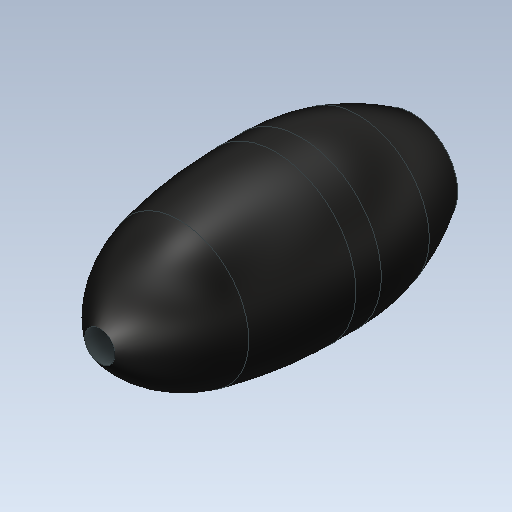
# Autodesk Inventor part: sail_weight
Saved by Autodesk Inventor 2020 (Build 240168000, 168)
## iProperties
Created: 2017-12-03
Part Number: sail_weight
Material: Lead
Document SubType Name: Modeling
Designer: stedrock
Density: 11.34 g/cm^3
Appearance: Lead
Mass: 409.157 g
Surface Area: 57.3985 cm^2
Volume: 36.0808 cm^3
Author: stedrock
Autodesk Inventor part; units mm, degrees
ref_plane "YZ Plane" through (0, 0, 0) normal (1, 0, 0) x (0, 1, 0)
ref_plane "XZ Plane" through (0, 0, 0) normal (0, 1, 0) x (-1, 0, 0)
ref_plane "XY Plane" through (0, 0, 0) normal (0, 0, 1) x (1, 0, 0)
sketch "Sketch1" plane through (0, 0, 0) normal (1, 0, 0) x (0, 1, 0)
  line L0 (0, 0) -> (0, 63)
  line L1 (0, 0) -> (9, 0)
  line L2 (15.9, 22) -> (15.9, 27)
  arc A0 (14.1466, 10.7593) -> (15.9, 22) centre (-21.0068, 22) ccw
  arc A1 (9, 0) -> (14.1466, 10.7593) centre (-27.5407, 24.0893) ccw
  arc A2 (15.9, 27) -> (15.9, 27) centre (-40077.1724, 27) ccw
  arc A3 (15.9, 27) -> (13.7227, 45.9678) centre (-67.8106, 27) ccw
  arc A4 (13.7227, 45.9678) -> (1.5995, 62.5596) centre (-11.8275, 40.0238) ccw
  arc A5 (1.5995, 62.5596) -> (0, 63) centre (0, 59.875) ccw
  dimension "d0" = 63
  dimension "d1" = 9
  dimension "d2" = 15.9
  dimension "d4" = 5
  dimension "d5" = 22
  constraints: 12 point on circle, 6 centre point, 6 end point, 6 tangent, 2 vertical, 1 horizontal, 1 line through centre, 1 point on line
  measures "d0" distance of L0.start L0.end
  measures "d1" distance of L0.start L1.end
  measures "d2" distance between parallel lines of L0 L2
  measures "d4" distance of L2.start L2.end
  measures "d5" distance from line of L1 L2.start
revolve "Revolution1" add sketch "Sketch1" angle 360 about axis through (0, 0, 0) along (0, 0, 1) contours L0 A5 A4 A3 L2 A0 A1 L1
sketch "Sketch2" plane through (0, 0, 0) normal (0, 0, 1) x (1, 0, 0)
  circle A0 centre (0, 0) radius 3
  dimension "d6" = 6
  constraints: 1 centre point, 1 coincident
  measures "d6" diameter of A0
extrude "hole" cut sketch "Sketch2" along normal through all
shell "Shell1" [suppressed]
split "Split1" [suppressed]
sketch "ribs" plane through (0, 0, 0) normal (1, 0, 0) x (0, 1, 0)
  line L0 (0, 0) -> (0, 68.6975) construction
  line L1 (0, 0) -> (23.2714, 0) construction
  line L2 (-0.6, 80.4959) -> (0.6, 80.4959)
  line L3 (0.6, 80.4959) -> (0.6, -19.5041)
  line L4 (0.6, -19.5041) -> (-0.6, -19.5041)
  line L5 (-0.6, -19.5041) -> (-0.6, 80.4959)
  line L6 (-0.6, 80.4959) -> (0.6, -19.5041) construction
  line L7 (0.6, 80.4959) -> (-0.6, -19.5041) construction
  line L8 (0, 0) -> (0, -28.2792) construction
  line L9 (-21.2582, -13.3041) -> (21.2582, -13.3041)
  line L10 (21.2582, -13.3041) -> (21.2582, -14.5041)
  line L11 (21.2582, -14.5041) -> (-21.2582, -14.5041)
  line L12 (-21.2582, -14.5041) -> (-21.2582, -13.3041)
  line L13 (-21.2582, -13.3041) -> (21.2582, -14.5041) construction
  line L14 (21.2582, -13.3041) -> (-21.2582, -14.5041) construction
  line L15 (0, 0) -> (34.6426, 0) construction
  line L16 (9.4, 80.4959) -> (10.6, 80.4959)
  line L17 (10.6, -19.5041) -> (9.4, -19.5041)
  line L18 (10, 0) -> (10, -28.2792) construction
  line L19 (10.6, 80.4959) -> (10.6, -19.5041)
  line L20 (9.4, -19.5041) -> (9.4, 80.4959)
  line L21 (9.4, 80.4959) -> (10.6, -19.5041) construction
  line L22 (10.6, 80.4959) -> (9.4, -19.5041) construction
  line L23 (19.4, 80.4959) -> (20.6, 80.4959)
  line L24 (20.6, -19.5041) -> (19.4, -19.5041)
  line L25 (20, 0) -> (20, -28.2792) construction
  line L26 (20.6, 80.4959) -> (20.6, -19.5041)
  line L27 (19.4, -19.5041) -> (19.4, 80.4959)
  line L28 (19.4, 80.4959) -> (20.6, -19.5041) construction
  line L29 (20.6, 80.4959) -> (19.4, -19.5041) construction
  line L30 (29.4, 80.4959) -> (30.6, 80.4959)
  line L31 (30.6, -19.5041) -> (29.4, -19.5041)
  line L32 (30, 0) -> (30, -28.2792) construction
  line L33 (30.6, 80.4959) -> (30.6, -19.5041)
  line L34 (29.4, -19.5041) -> (29.4, 80.4959)
  line L35 (29.4, 80.4959) -> (30.6, -19.5041) construction
  line L36 (30.6, 80.4959) -> (29.4, -19.5041) construction
  line L37 (39.4, 80.4959) -> (40.6, 80.4959)
  line L38 (40.6, -19.5041) -> (39.4, -19.5041)
  line L39 (40, 0) -> (40, -28.2792) construction
  line L40 (40.6, 80.4959) -> (40.6, -19.5041)
  line L41 (39.4, -19.5041) -> (39.4, 80.4959)
  line L42 (39.4, 80.4959) -> (40.6, -19.5041) construction
  line L43 (40.6, 80.4959) -> (39.4, -19.5041) construction
  line L44 (21.2582, -3.3041) -> (21.2582, -4.5041)
  line L45 (21.2582, -4.5041) -> (-21.2582, -4.5041)
  line L46 (-21.2582, -3.3041) -> (21.2582, -3.3041)
  line L47 (-21.2582, -3.3041) -> (21.2582, -4.5041) construction
  line L48 (21.2582, -3.3041) -> (-21.2582, -4.5041) construction
  line L49 (-21.2582, -4.5041) -> (-21.2582, -3.3041)
  line L50 (21.2582, 6.6959) -> (21.2582, 5.4959)
  line L51 (21.2582, 5.4959) -> (-21.2582, 5.4959)
  line L52 (-21.2582, 6.6959) -> (21.2582, 6.6959)
  line L53 (-21.2582, 6.6959) -> (21.2582, 5.4959) construction
  line L54 (21.2582, 6.6959) -> (-21.2582, 5.4959) construction
  line L55 (-21.2582, 5.4959) -> (-21.2582, 6.6959)
  line L56 (21.2582, 16.6959) -> (21.2582, 15.4959)
  line L57 (21.2582, 15.4959) -> (-21.2582, 15.4959)
  line L58 (-21.2582, 16.6959) -> (21.2582, 16.6959)
  line L59 (-21.2582, 16.6959) -> (21.2582, 15.4959) construction
  line L60 (21.2582, 16.6959) -> (-21.2582, 15.4959) construction
  line L61 (-21.2582, 15.4959) -> (-21.2582, 16.6959)
  line L62 (21.2582, 26.6959) -> (21.2582, 25.4959)
  line L63 (21.2582, 25.4959) -> (-21.2582, 25.4959)
  line L64 (-21.2582, 26.6959) -> (21.2582, 26.6959)
  line L65 (-21.2582, 26.6959) -> (21.2582, 25.4959) construction
  line L66 (21.2582, 26.6959) -> (-21.2582, 25.4959) construction
  line L67 (-21.2582, 25.4959) -> (-21.2582, 26.6959)
  line L68 (21.2582, 36.6959) -> (21.2582, 35.4959)
  line L69 (21.2582, 35.4959) -> (-21.2582, 35.4959)
  line L70 (-21.2582, 36.6959) -> (21.2582, 36.6959)
  line L71 (-21.2582, 36.6959) -> (21.2582, 35.4959) construction
  line L72 (21.2582, 36.6959) -> (-21.2582, 35.4959) construction
  line L73 (-21.2582, 35.4959) -> (-21.2582, 36.6959)
  line L74 (21.2582, 46.6959) -> (21.2582, 45.4959)
  line L75 (21.2582, 45.4959) -> (-21.2582, 45.4959)
  line L76 (-21.2582, 46.6959) -> (21.2582, 46.6959)
  line L77 (-21.2582, 46.6959) -> (21.2582, 45.4959) construction
  line L78 (21.2582, 46.6959) -> (-21.2582, 45.4959) construction
  line L79 (-21.2582, 45.4959) -> (-21.2582, 46.6959)
  line L80 (21.2582, 56.6959) -> (21.2582, 55.4959)
  line L81 (21.2582, 55.4959) -> (-21.2582, 55.4959)
  line L82 (-21.2582, 56.6959) -> (21.2582, 56.6959)
  line L83 (-21.2582, 56.6959) -> (21.2582, 55.4959) construction
  line L84 (21.2582, 56.6959) -> (-21.2582, 55.4959) construction
  line L85 (-21.2582, 55.4959) -> (-21.2582, 56.6959)
  line L86 (21.2582, 66.6959) -> (21.2582, 65.4959)
  line L87 (21.2582, 65.4959) -> (-21.2582, 65.4959)
  line L88 (-21.2582, 66.6959) -> (21.2582, 66.6959)
  line L89 (-21.2582, 66.6959) -> (21.2582, 65.4959) construction
  line L90 (21.2582, 66.6959) -> (-21.2582, 65.4959) construction
  line L91 (-21.2582, 65.4959) -> (-21.2582, 66.6959)
  line L92 (21.2582, 76.6959) -> (21.2582, 75.4959)
  line L93 (21.2582, 75.4959) -> (-21.2582, 75.4959)
  line L94 (-21.2582, 76.6959) -> (21.2582, 76.6959)
  line L95 (-21.2582, 76.6959) -> (21.2582, 75.4959) construction
  line L96 (21.2582, 76.6959) -> (-21.2582, 75.4959) construction
  line L97 (-21.2582, 75.4959) -> (-21.2582, 76.6959)
  line L98 (21.2582, 86.6959) -> (21.2582, 85.4959)
  line L99 (21.2582, 85.4959) -> (-21.2582, 85.4959)
  line L100 (-21.2582, 86.6959) -> (21.2582, 86.6959)
  line L101 (-21.2582, 86.6959) -> (21.2582, 85.4959) construction
  line L102 (21.2582, 86.6959) -> (-21.2582, 85.4959) construction
  line L103 (-21.2582, 85.4959) -> (-21.2582, 86.6959)
  line L104 (21.2582, 96.6959) -> (21.2582, 95.4959)
  line L105 (21.2582, 95.4959) -> (-21.2582, 95.4959)
  line L106 (-21.2582, 96.6959) -> (21.2582, 96.6959)
  line L107 (-21.2582, 96.6959) -> (21.2582, 95.4959) construction
  line L108 (21.2582, 96.6959) -> (-21.2582, 95.4959) construction
  line L109 (-21.2582, 95.4959) -> (-21.2582, 96.6959)
  line L110 (21.2582, 106.6959) -> (21.2582, 105.4959)
  line L111 (21.2582, 105.4959) -> (-21.2582, 105.4959)
  line L112 (-21.2582, 106.6959) -> (21.2582, 106.6959)
  line L113 (-21.2582, 106.6959) -> (21.2582, 105.4959) construction
  line L114 (21.2582, 106.6959) -> (-21.2582, 105.4959) construction
  line L115 (-21.2582, 105.4959) -> (-21.2582, 106.6959)
  line L116 (21.2582, 116.6959) -> (21.2582, 115.4959)
  line L117 (21.2582, 115.4959) -> (-21.2582, 115.4959)
  line L118 (-21.2582, 116.6959) -> (21.2582, 116.6959)
  line L119 (-21.2582, 116.6959) -> (21.2582, 115.4959) construction
  line L120 (21.2582, 116.6959) -> (-21.2582, 115.4959) construction
  line L121 (-21.2582, 115.4959) -> (-21.2582, 116.6959)
  line L122 (21.2582, 126.6959) -> (21.2582, 125.4959)
  line L123 (21.2582, 125.4959) -> (-21.2582, 125.4959)
  line L124 (-21.2582, 126.6959) -> (21.2582, 126.6959)
  line L125 (-21.2582, 126.6959) -> (21.2582, 125.4959) construction
  line L126 (21.2582, 126.6959) -> (-21.2582, 125.4959) construction
  line L127 (-21.2582, 125.4959) -> (-21.2582, 126.6959)
  line L128 (21.2582, 136.6959) -> (21.2582, 135.4959)
  line L129 (21.2582, 135.4959) -> (-21.2582, 135.4959)
  line L130 (-21.2582, 136.6959) -> (21.2582, 136.6959)
  line L131 (-21.2582, 136.6959) -> (21.2582, 135.4959) construction
  line L132 (21.2582, 136.6959) -> (-21.2582, 135.4959) construction
  line L133 (-21.2582, 135.4959) -> (-21.2582, 136.6959)
  line L134 (21.2582, 146.6959) -> (21.2582, 145.4959)
  line L135 (21.2582, 145.4959) -> (-21.2582, 145.4959)
  line L136 (-21.2582, 146.6959) -> (21.2582, 146.6959)
  line L137 (-21.2582, 146.6959) -> (21.2582, 145.4959) construction
  line L138 (21.2582, 146.6959) -> (-21.2582, 145.4959) construction
  line L139 (-21.2582, 145.4959) -> (-21.2582, 146.6959)
  line L140 (21.2582, 156.6959) -> (21.2582, 155.4959)
  line L141 (21.2582, 155.4959) -> (-21.2582, 155.4959)
  line L142 (-21.2582, 156.6959) -> (21.2582, 156.6959)
  line L143 (-21.2582, 156.6959) -> (21.2582, 155.4959) construction
  line L144 (21.2582, 156.6959) -> (-21.2582, 155.4959) construction
  line L145 (-21.2582, 155.4959) -> (-21.2582, 156.6959)
  line L146 (-9.4, 80.4959) -> (-9.4, -19.5041)
  line L147 (-10.6, 80.4959) -> (-9.4, 80.4959)
  line L148 (-10.6, 80.4959) -> (-9.4, -19.5041) construction
  line L149 (-10.6, -19.5041) -> (-10.6, 80.4959)
  line L150 (-9.4, 80.4959) -> (-10.6, -19.5041) construction
  line L151 (-9.4, -19.5041) -> (-10.6, -19.5041)
  line L152 (-10, 0) -> (-10, -28.2792) construction
  line L153 (-19.4, 80.4959) -> (-19.4, -19.5041)
  line L154 (-20.6, 80.4959) -> (-19.4, 80.4959)
  line L155 (-20.6, 80.4959) -> (-19.4, -19.5041) construction
  line L156 (-20.6, -19.5041) -> (-20.6, 80.4959)
  line L157 (-19.4, 80.4959) -> (-20.6, -19.5041) construction
  line L158 (-19.4, -19.5041) -> (-20.6, -19.5041)
  line L159 (-20, 0) -> (-20, -28.2792) construction
  line L160 (-29.4, 80.4959) -> (-29.4, -19.5041)
  line L161 (-30.6, 80.4959) -> (-29.4, 80.4959)
  line L162 (-30.6, 80.4959) -> (-29.4, -19.5041) construction
  line L163 (-30.6, -19.5041) -> (-30.6, 80.4959)
  line L164 (-29.4, 80.4959) -> (-30.6, -19.5041) construction
  line L165 (-29.4, -19.5041) -> (-30.6, -19.5041)
  line L166 (-30, 0) -> (-30, -28.2792) construction
  line L167 (-39.4, 80.4959) -> (-39.4, -19.5041)
  line L168 (-40.6, 80.4959) -> (-39.4, 80.4959)
  line L169 (-40.6, 80.4959) -> (-39.4, -19.5041) construction
  line L170 (-40.6, -19.5041) -> (-40.6, 80.4959)
  line L171 (-39.4, 80.4959) -> (-40.6, -19.5041) construction
  line L172 (-39.4, -19.5041) -> (-40.6, -19.5041)
  line L173 (-40, 0) -> (-40, -28.2792) construction
  point P0 (0, 30.4959)
  point P1 (0, -13.9041)
  point P2 (10, -13.9041)
  point P3 (20, -13.9041)
  point P4 (30, -13.9041)
  point P5 (40, -13.9041)
  point P6 (-10, -13.9041)
  point P7 (-20, -13.9041)
  point P8 (-30, -13.9041)
  point P9 (-40, -13.9041)
  dimension "d10" = 100
  dimension "d11" = 1.2
  dimension "d12" = 1.2
  dimension "d13" = 5
  dimension "d16" = 10
  dimension "d30" = 10
  dimension "d39" = 10
  constraints: 348 end point, 10 point on line, 6 horizontal, 4 midpoint, 4 parallel, 3 vertical, 2 perpendicular, 282 other
  measures "d10" distance of L4.end L2.start
  measures "d11" distance of L3.end L4.end
  measures "d12" distance of L9.end L10.end
  measures "d13" distance between parallel lines of L4 L11
  measures "d16" distance of L2.start L16.start
  measures "d30" distance of L10.end L44.end
  measures "d39" distance of L2.end L146.start
extrude "ribs Extrusion" [suppressed]
sketch "pins" plane through (0, 0, 0) normal (1, 0, 0) x (0, 1, 0)
  circle A0 centre (-6.5516, 52.6251) radius 1.5
  circle A1 centre (-6.5516, 52.6251) radius 3
  circle A2 centre (6.628, 52.7726) radius 1.5
  circle A3 centre (6.628, 52.7726) radius 3
  circle A4 centre (6.7755, 3.9597) radius 1.5
  circle A5 centre (6.7755, 3.9597) radius 3
  circle A6 centre (-6.754, 3.939) radius 3
  circle A7 centre (-6.754, 3.939) radius 1.5
  point P0 (0, 0)
  dimension "d44" = 3
  dimension "d45" = 6
  dimension "d46" = 3
  dimension "d47" = 6
  dimension "d48" = 3
  dimension "d49" = 6
  dimension "d50" = 3
  dimension "d51" = 6
  constraints: 8 centre point, 4 coincident
  measures "d44" diameter of A0
  measures "d45" diameter of A1
  measures "d46" diameter of A2
  measures "d47" diameter of A3
  measures "d48" diameter of A4
  measures "d49" diameter of A5
  measures "d50" diameter of A7
  measures "d51" diameter of A6
extrude "pins Extrusion" [suppressed]
mirror "Mirror1" [suppressed]
equation "\"d9\" = wall"
equation "\"d11\" = wall"
equation "\"d12\" = wall"
equation "\"d16\" = ribs"
equation "\"d30\" = ribs"
equation "\"d39\" = ribs"
equation "\"wall\" = 1.2"
equation "\"ribs\" = 10"
body "Solid1"
